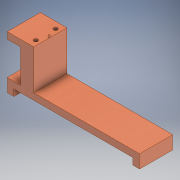
# Autodesk Inventor part: Part1
Saved by Autodesk Inventor 2020 (Build 240168000, 168)
## iProperties
Created: 2021-11-29
Part Number: Part1
Material: Wood (Walnut)
Document SubType Name: Modeling
Designer: Emrah BAYRAM
Density: 0.55 g/cm^3
Appearance: Walnut - Natural Polished
Mass: 13297.4 g
Surface Area: 10734.2 cm^2
Volume: 24177.1 cm^3
Author: Emrah BAYRAM
Autodesk Inventor part; units mm, degrees
ref_plane "YZ Plane" through (0, 0, 0) normal (1, 0, 0) x (0, 1, 0)
ref_plane "XZ Plane" through (0, 0, 0) normal (0, 1, 0) x (-1, 0, 0)
ref_plane "XY Plane" through (0, 0, 0) normal (0, 0, 1) x (1, 0, 0)
sketch "Sketch1" plane through (0, 0, 0) normal (0, 0, 1) x (1, 0, 0)
  line L0 (0, 0) -> (200, 0)
  line L1 (200, 0) -> (200, -300)
  line L2 (200, -300) -> (1000, -300)
  line L3 (1000, -300) -> (1000, -400)
  line L4 (1000, -400) -> (950, -400)
  line L5 (950, -400) -> (950, -350)
  line L6 (950, -350) -> (50, -350)
  line L7 (50, -350) -> (50, -400)
  line L8 (0, -400) -> (50, -400)
  line L9 (950, -400) -> (1000, -400)
  line L10 (0, -300) -> (100, -300)
  line L11 (100, -300) -> (100, -50)
  line L12 (100, -50) -> (0, -50)
  line L13 (0, 0) -> (0, -50)
  line L14 (0, -300) -> (0, -400)
  dimension "d0" = 200
  dimension "d1" = 300
  dimension "d2" = 800
  dimension "d3" = 100
  dimension "d41" = 50
  dimension "d42" = 900
  dimension "d43" = 100
  dimension "d44" = 250
  constraints: 30 end point, 14 perpendicular, 2 point on line, 2 vertical, 1 horizontal
  measures "d0" distance of L0.start L0.end
  measures "d1" distance of L0.end L1.end
  measures "d2" distance of L1.end L2.end
  measures "d3" distance of L2.end L3.end
  measures "d41" distance of L3.end L4.end
  measures "d42" distance of L5.end L6.end
  measures "d43" distance of L10.start L10.end
  measures "d44" distance of L10.end L11.end
extrude "Extrusion1" add sketch "Sketch1" along normal blind 250
sketch "Sketch2" plane through (0, 0, 0) normal (0, 1, 0) x (1, 0, 0)
  line L0 (200, 0) -> (0, 0) projected
  line L1 (200, 0) -> (150, 0)
  line L2 (200, -250) -> (0, -250) projected
  line L3 (200, -250) -> (150, -250)
  circle A0 centre (165, -50) radius 15
  circle A1 centre (165, -200) radius 15
  line L4 (200, 0) -> (200, -250) projected
  dimension "d9" = 50
  dimension "d11" = 30
  dimension "d12" = 30
  dimension "d36" = 35
  dimension "d37" = 35
  constraints: 4 end point, 2 centre point, 2 point on line
  measures "d9" distance of L2.start L3.end
  measures "d11" diameter of A0
  measures "d12" diameter of A1
  measures "d36" distance from line of L4 A1.centre
  measures "d37" distance from line of L4 A0.centre
sketch "Sketch4" plane through (0, 0, 0) normal (0, 1, 0) x (1, 0, 0)
  line L0 (200, 0) -> (200, -250) projected
  line L1 (200, -125) -> (192.5, -125)
  circle A0 centre (192.5, -125) radius 7.5
  point P0 (0, 0)
  dimension "d38" = 7.5
  constraints: 2 end point, 1 centre point, 1 coincident, 1 midpoint, 1 perpendicular
  measures "d38" distance of L1.start L1.end
extrude "Extrusion7" add sketch "Sketch4" along normal blind 10
extrude "Extrusion8" cut sketch "Sketch2" against normal blind 30
body "Solid1"
